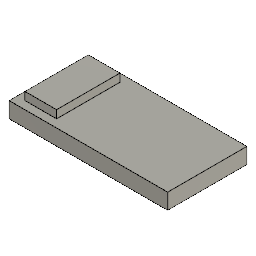
machine arm v5 (Autodesk Fusion 360 design; units mm, degrees)
Autodesk Fusion 360 part; units mm, degrees
sketch "machine arm" plane through (0, 0, 0) normal (0, 0, 1) x (1, 0, 0)
  line L0 (-50, -25) -> (50, -25)
  line L1 (50, -25) -> (50, 25)
  line L2 (50, 25) -> (-50, 25)
  line L3 (-50, 25) -> (-50, -25)
  line L4 (-50, -25) -> (50, 25) construction
  line L5 (50, -25) -> (-50, 25) construction
  dimension "d1" = 100
  dimension "d2" = 50
  constraint horizontal L0
  constraint perpendicular L0 L1
  constraint parallel L0 L2
  constraint parallel L1 L3
  constraint coincident L4 origin
  constraint coincident L5 origin
  measures "d1" distance of L1.end L2.end
  measures "d2" distance of L0.end L1.end
extrude "Extrude1" add sketch "machine arm" along normal blind 10
sketch "socket" plane through (0, 0, 0) normal (0, 0, -1) x (1, 0, 0)
  line L0 (-50, 25) -> (-50, -25)
  line L1 (-50, -25) -> (50, -25)
  line L2 (50, -25) -> (50, 25)
  line L3 (50, 25) -> (-50, 25)
  line L4 (47.5, 10) -> (32.5, 10)
  line L5 (32.5, 10) -> (32.5, -10)
  line L6 (32.5, -10) -> (47.5, -10)
  line L7 (47.5, -10) -> (47.5, 10)
  line L8 (47.5, 10) -> (32.5, -10) construction
  line L9 (32.5, 10) -> (47.5, -10) construction
  point P0 (40, 0)
  dimension "d5" = 15
  dimension "d6" = 20
  constraint horizontal L4
  constraint perpendicular L4 L5
  constraint parallel L4 L6
  constraint parallel L5 L7
  constraint coincident L8 P0
  constraint coincident L9 P0
  measures "d5" distance of L5.end L6.end
  measures "d6" distance of L4.end L5.end
extrude "Extrude2" cut sketch "socket" against normal blind 5 contours L4 L5 L6 L7
sketch "Sketch3" plane through (0, 0, 10) normal (0, 0, 1) x (-1, 0, 0)
  line L0 (50, -25) -> (50, 25)
  line L1 (50, 25) -> (-50, 25)
  line L2 (-50, 25) -> (-50, -25)
  line L3 (-50, -25) -> (50, -25)
  line L4 (25, -20) -> (45, -20)
  line L5 (45, -20) -> (45, 20)
  line L6 (45, 20) -> (25, 20)
  line L7 (25, 20) -> (25, -20)
  point P0 (25, -20)
  constraint horizontal L4
  constraint vertical L5
  constraint horizontal L6
  constraint vertical L7
  constraint coincident P0 L4.start
extrude "Extrude3" add sketch "Sketch3" along normal blind 5 contours L4 L5 L6 L7
